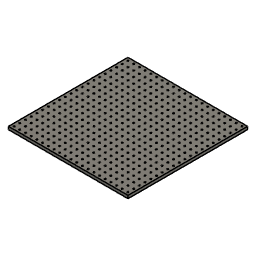
Robot base (Autodesk Fusion 360 design; units mm, degrees)
Autodesk Fusion 360 part; units mm, degrees
sketch "Sketch1" plane through (0, 0, 0) normal (0, 1, 0) x (1, 0, 0) in component "RobotPlatformBase"
  line L0 (-105, 105) -> (105, 105)
  line L1 (105, 105) -> (105, -105)
  line L2 (105, -105) -> (-105, -105)
  line L3 (-105, -105) -> (-105, 105)
  line L4 (-105, -105) -> (105, 105) construction
  dimension "d1" = 210
  constraint horizontal L0
  constraint vertical L1
  constraint horizontal L2
  constraint vertical L3
  constraint midpoint origin L4
  constraint equal L0 L3
  measures "d1" distance of L0.start L0.end
extrude "Extrude1" add sketch "Sketch1" along normal blind 5 in component "RobotPlatformBase"
sketch "Sketch2" plane through (0, 5, 0) normal (0, 1, 0) x (-1, 0, 0) in component "RobotPlatformBase"
  line L0 (105, 105) -> (-105, 105)
  line L1 (-105, 105) -> (-105, -105)
  line L2 (-105, -105) -> (105, -105)
  line L3 (105, -105) -> (105, 105)
  circle A0 centre (100, -100) radius 1.35
  circle A1 centre (90, -100) radius 1.35
  circle A2 centre (80, -100) radius 1.35
  circle A3 centre (70, -100) radius 1.35
  circle A4 centre (60, -100) radius 1.35
  circle A5 centre (50, -100) radius 1.35
  circle A6 centre (40, -100) radius 1.35
  circle A7 centre (30, -100) radius 1.35
  circle A8 centre (20, -100) radius 1.35
  circle A9 centre (10, -100) radius 1.35
  circle A10 centre (0, -100) radius 1.35
  circle A11 centre (-10, -100) radius 1.35
  circle A12 centre (-20, -100) radius 1.35
  circle A13 centre (-30, -100) radius 1.35
  circle A14 centre (-40, -100) radius 1.35
  circle A15 centre (-50, -100) radius 1.35
  circle A16 centre (-60, -100) radius 1.35
  circle A17 centre (-70, -100) radius 1.35
  circle A18 centre (-80, -100) radius 1.35
  circle A19 centre (-90, -100) radius 1.35
  circle A20 centre (100, -90) radius 1.35
  circle A21 centre (90, -90) radius 1.35
  circle A22 centre (80, -90) radius 1.35
  circle A23 centre (70, -90) radius 1.35
  circle A24 centre (60, -90) radius 1.35
  circle A25 centre (50, -90) radius 1.35
  circle A26 centre (40, -90) radius 1.35
  circle A27 centre (30, -90) radius 1.35
  circle A28 centre (20, -90) radius 1.35
  circle A29 centre (10, -90) radius 1.35
  circle A30 centre (0, -90) radius 1.35
  circle A31 centre (-10, -90) radius 1.35
  circle A32 centre (-20, -90) radius 1.35
  circle A33 centre (-30, -90) radius 1.35
  circle A34 centre (-40, -90) radius 1.35
  circle A35 centre (-50, -90) radius 1.35
  circle A36 centre (-60, -90) radius 1.35
  circle A37 centre (-70, -90) radius 1.35
  circle A38 centre (-80, -90) radius 1.35
  circle A39 centre (-90, -90) radius 1.35
  circle A40 centre (100, -80) radius 1.35
  circle A41 centre (90, -80) radius 1.35
  circle A42 centre (80, -80) radius 1.35
  circle A43 centre (70, -80) radius 1.35
  circle A44 centre (60, -80) radius 1.35
  circle A45 centre (50, -80) radius 1.35
  circle A46 centre (40, -80) radius 1.35
  circle A47 centre (30, -80) radius 1.35
  circle A48 centre (20, -80) radius 1.35
  circle A49 centre (10, -80) radius 1.35
  circle A50 centre (0, -80) radius 1.35
  circle A51 centre (-10, -80) radius 1.35
  circle A52 centre (-20, -80) radius 1.35
  circle A53 centre (-30, -80) radius 1.35
  circle A54 centre (-40, -80) radius 1.35
  circle A55 centre (-50, -80) radius 1.35
  circle A56 centre (-60, -80) radius 1.35
  circle A57 centre (-70, -80) radius 1.35
  circle A58 centre (-80, -80) radius 1.35
  circle A59 centre (-90, -80) radius 1.35
  circle A60 centre (100, -70) radius 1.35
  circle A61 centre (90, -70) radius 1.35
  circle A62 centre (80, -70) radius 1.35
  circle A63 centre (70, -70) radius 1.35
  circle A64 centre (60, -70) radius 1.35
  circle A65 centre (50, -70) radius 1.35
  circle A66 centre (40, -70) radius 1.35
  circle A67 centre (30, -70) radius 1.35
  circle A68 centre (20, -70) radius 1.35
  circle A69 centre (10, -70) radius 1.35
  circle A70 centre (0, -70) radius 1.35
  circle A71 centre (-10, -70) radius 1.35
  circle A72 centre (-20, -70) radius 1.35
  circle A73 centre (-30, -70) radius 1.35
  circle A74 centre (-40, -70) radius 1.35
  circle A75 centre (-50, -70) radius 1.35
  circle A76 centre (-60, -70) radius 1.35
  circle A77 centre (-70, -70) radius 1.35
  circle A78 centre (-80, -70) radius 1.35
  circle A79 centre (-90, -70) radius 1.35
  circle A80 centre (100, -60) radius 1.35
  circle A81 centre (90, -60) radius 1.35
  circle A82 centre (80, -60) radius 1.35
  circle A83 centre (70, -60) radius 1.35
  circle A84 centre (60, -60) radius 1.35
  circle A85 centre (50, -60) radius 1.35
  circle A86 centre (40, -60) radius 1.35
  circle A87 centre (30, -60) radius 1.35
  circle A88 centre (20, -60) radius 1.35
  circle A89 centre (10, -60) radius 1.35
  circle A90 centre (0, -60) radius 1.35
  circle A91 centre (-10, -60) radius 1.35
  circle A92 centre (-20, -60) radius 1.35
  circle A93 centre (-30, -60) radius 1.35
  circle A94 centre (-40, -60) radius 1.35
  circle A95 centre (-50, -60) radius 1.35
  circle A96 centre (-60, -60) radius 1.35
  circle A97 centre (-70, -60) radius 1.35
  circle A98 centre (-80, -60) radius 1.35
  circle A99 centre (-90, -60) radius 1.35
  circle A100 centre (100, -50) radius 1.35
  circle A101 centre (90, -50) radius 1.35
  circle A102 centre (80, -50) radius 1.35
  circle A103 centre (70, -50) radius 1.35
  circle A104 centre (60, -50) radius 1.35
  circle A105 centre (50, -50) radius 1.35
  circle A106 centre (40, -50) radius 1.35
  circle A107 centre (30, -50) radius 1.35
  circle A108 centre (20, -50) radius 1.35
  circle A109 centre (10, -50) radius 1.35
  circle A110 centre (0, -50) radius 1.35
  circle A111 centre (-10, -50) radius 1.35
  circle A112 centre (-20, -50) radius 1.35
  circle A113 centre (-30, -50) radius 1.35
  circle A114 centre (-40, -50) radius 1.35
  circle A115 centre (-50, -50) radius 1.35
  circle A116 centre (-60, -50) radius 1.35
  circle A117 centre (-70, -50) radius 1.35
  circle A118 centre (-80, -50) radius 1.35
  circle A119 centre (-90, -50) radius 1.35
  circle A120 centre (100, -40) radius 1.35
  circle A121 centre (90, -40) radius 1.35
  circle A122 centre (80, -40) radius 1.35
  circle A123 centre (70, -40) radius 1.35
  circle A124 centre (60, -40) radius 1.35
  circle A125 centre (50, -40) radius 1.35
  circle A126 centre (40, -40) radius 1.35
  circle A127 centre (30, -40) radius 1.35
  circle A128 centre (20, -40) radius 1.35
  circle A129 centre (10, -40) radius 1.35
  circle A130 centre (0, -40) radius 1.35
  circle A131 centre (-10, -40) radius 1.35
  circle A132 centre (-20, -40) radius 1.35
  circle A133 centre (-30, -40) radius 1.35
  circle A134 centre (-40, -40) radius 1.35
  circle A135 centre (-50, -40) radius 1.35
  circle A136 centre (-60, -40) radius 1.35
  circle A137 centre (-70, -40) radius 1.35
  circle A138 centre (-80, -40) radius 1.35
  circle A139 centre (-90, -40) radius 1.35
  circle A140 centre (100, -30) radius 1.35
  circle A141 centre (90, -30) radius 1.35
  circle A142 centre (80, -30) radius 1.35
  circle A143 centre (70, -30) radius 1.35
  circle A144 centre (60, -30) radius 1.35
  circle A145 centre (50, -30) radius 1.35
  circle A146 centre (40, -30) radius 1.35
  circle A147 centre (30, -30) radius 1.35
  circle A148 centre (20, -30) radius 1.35
  circle A149 centre (10, -30) radius 1.35
  circle A150 centre (0, -30) radius 1.35
  circle A151 centre (-10, -30) radius 1.35
  circle A152 centre (-20, -30) radius 1.35
  circle A153 centre (-30, -30) radius 1.35
  circle A154 centre (-40, -30) radius 1.35
  circle A155 centre (-50, -30) radius 1.35
  circle A156 centre (-60, -30) radius 1.35
  circle A157 centre (-70, -30) radius 1.35
  circle A158 centre (-80, -30) radius 1.35
  circle A159 centre (-90, -30) radius 1.35
  circle A160 centre (100, -20) radius 1.35
  circle A161 centre (90, -20) radius 1.35
  circle A162 centre (80, -20) radius 1.35
  circle A163 centre (70, -20) radius 1.35
  circle A164 centre (60, -20) radius 1.35
  circle A165 centre (50, -20) radius 1.35
  circle A166 centre (40, -20) radius 1.35
  circle A167 centre (30, -20) radius 1.35
  circle A168 centre (20, -20) radius 1.35
  circle A169 centre (10, -20) radius 1.35
  circle A170 centre (0, -20) radius 1.35
  circle A171 centre (-10, -20) radius 1.35
  circle A172 centre (-20, -20) radius 1.35
  circle A173 centre (-30, -20) radius 1.35
  circle A174 centre (-40, -20) radius 1.35
  circle A175 centre (-50, -20) radius 1.35
  circle A176 centre (-60, -20) radius 1.35
  circle A177 centre (-70, -20) radius 1.35
  circle A178 centre (-80, -20) radius 1.35
  circle A179 centre (-90, -20) radius 1.35
  circle A180 centre (100, -10) radius 1.35
  circle A181 centre (90, -10) radius 1.35
  circle A182 centre (80, -10) radius 1.35
  circle A183 centre (70, -10) radius 1.35
  circle A184 centre (60, -10) radius 1.35
  circle A185 centre (50, -10) radius 1.35
  circle A186 centre (40, -10) radius 1.35
  circle A187 centre (30, -10) radius 1.35
  circle A188 centre (20, -10) radius 1.35
  circle A189 centre (10, -10) radius 1.35
  circle A190 centre (0, -10) radius 1.35
  circle A191 centre (-10, -10) radius 1.35
  circle A192 centre (-20, -10) radius 1.35
  circle A193 centre (-30, -10) radius 1.35
  circle A194 centre (-40, -10) radius 1.35
  circle A195 centre (-50, -10) radius 1.35
  circle A196 centre (-60, -10) radius 1.35
  circle A197 centre (-70, -10) radius 1.35
  circle A198 centre (-80, -10) radius 1.35
  circle A199 centre (-90, -10) radius 1.35
  circle A200 centre (100, 0) radius 1.35
  circle A201 centre (90, 0) radius 1.35
  circle A202 centre (80, 0) radius 1.35
  circle A203 centre (70, 0) radius 1.35
  circle A204 centre (60, 0) radius 1.35
  circle A205 centre (50, 0) radius 1.35
  circle A206 centre (40, 0) radius 1.35
  circle A207 centre (30, 0) radius 1.35
  circle A208 centre (20, 0) radius 1.35
  circle A209 centre (10, 0) radius 1.35
  circle A210 centre (0, 0) radius 1.35
  circle A211 centre (-10, 0) radius 1.35
  circle A212 centre (-20, 0) radius 1.35
  circle A213 centre (-30, 0) radius 1.35
  circle A214 centre (-40, 0) radius 1.35
  circle A215 centre (-50, 0) radius 1.35
  circle A216 centre (-60, 0) radius 1.35
  circle A217 centre (-70, 0) radius 1.35
  circle A218 centre (-80, 0) radius 1.35
  circle A219 centre (-90, 0) radius 1.35
  circle A220 centre (100, 10) radius 1.35
  circle A221 centre (90, 10) radius 1.35
  circle A222 centre (80, 10) radius 1.35
  circle A223 centre (70, 10) radius 1.35
  circle A224 centre (60, 10) radius 1.35
  circle A225 centre (50, 10) radius 1.35
  circle A226 centre (40, 10) radius 1.35
  circle A227 centre (30, 10) radius 1.35
  circle A228 centre (20, 10) radius 1.35
  circle A229 centre (10, 10) radius 1.35
  circle A230 centre (0, 10) radius 1.35
  circle A231 centre (-10, 10) radius 1.35
  circle A232 centre (-20, 10) radius 1.35
  circle A233 centre (-30, 10) radius 1.35
  circle A234 centre (-40, 10) radius 1.35
  circle A235 centre (-50, 10) radius 1.35
  circle A236 centre (-60, 10) radius 1.35
  circle A237 centre (-70, 10) radius 1.35
  circle A238 centre (-80, 10) radius 1.35
  circle A239 centre (-90, 10) radius 1.35
  circle A240 centre (100, 20) radius 1.35
  circle A241 centre (90, 20) radius 1.35
  circle A242 centre (80, 20) radius 1.35
  circle A243 centre (70, 20) radius 1.35
  circle A244 centre (60, 20) radius 1.35
  circle A245 centre (50, 20) radius 1.35
  circle A246 centre (40, 20) radius 1.35
  circle A247 centre (30, 20) radius 1.35
  circle A248 centre (20, 20) radius 1.35
  circle A249 centre (10, 20) radius 1.35
  circle A250 centre (0, 20) radius 1.35
  circle A251 centre (-10, 20) radius 1.35
  circle A252 centre (-20, 20) radius 1.35
  circle A253 centre (-30, 20) radius 1.35
  circle A254 centre (-40, 20) radius 1.35
  circle A255 centre (-50, 20) radius 1.35
  circle A256 centre (-60, 20) radius 1.35
  circle A257 centre (-70, 20) radius 1.35
  circle A258 centre (-80, 20) radius 1.35
  circle A259 centre (-90, 20) radius 1.35
  circle A260 centre (100, 30) radius 1.35
  circle A261 centre (90, 30) radius 1.35
  circle A262 centre (80, 30) radius 1.35
  circle A263 centre (70, 30) radius 1.35
  circle A264 centre (60, 30) radius 1.35
  circle A265 centre (50, 30) radius 1.35
  circle A266 centre (40, 30) radius 1.35
  circle A267 centre (30, 30) radius 1.35
  circle A268 centre (20, 30) radius 1.35
  circle A269 centre (10, 30) radius 1.35
  circle A270 centre (0, 30) radius 1.35
  circle A271 centre (-10, 30) radius 1.35
  circle A272 centre (-20, 30) radius 1.35
  circle A273 centre (-30, 30) radius 1.35
  circle A274 centre (-40, 30) radius 1.35
  circle A275 centre (-50, 30) radius 1.35
  circle A276 centre (-60, 30) radius 1.35
  circle A277 centre (-70, 30) radius 1.35
  circle A278 centre (-80, 30) radius 1.35
  circle A279 centre (-90, 30) radius 1.35
  circle A280 centre (100, 40) radius 1.35
  circle A281 centre (90, 40) radius 1.35
  circle A282 centre (80, 40) radius 1.35
  circle A283 centre (70, 40) radius 1.35
  circle A284 centre (60, 40) radius 1.35
  circle A285 centre (50, 40) radius 1.35
  circle A286 centre (40, 40) radius 1.35
  circle A287 centre (30, 40) radius 1.35
  circle A288 centre (20, 40) radius 1.35
  circle A289 centre (10, 40) radius 1.35
  circle A290 centre (0, 40) radius 1.35
  circle A291 centre (-10, 40) radius 1.35
  circle A292 centre (-20, 40) radius 1.35
  circle A293 centre (-30, 40) radius 1.35
  circle A294 centre (-40, 40) radius 1.35
  circle A295 centre (-50, 40) radius 1.35
  circle A296 centre (-60, 40) radius 1.35
  circle A297 centre (-70, 40) radius 1.35
  circle A298 centre (-80, 40) radius 1.35
  circle A299 centre (-90, 40) radius 1.35
  circle A300 centre (100, 50) radius 1.35
  circle A301 centre (90, 50) radius 1.35
  circle A302 centre (80, 50) radius 1.35
  circle A303 centre (70, 50) radius 1.35
  circle A304 centre (60, 50) radius 1.35
  circle A305 centre (50, 50) radius 1.35
  circle A306 centre (40, 50) radius 1.35
  circle A307 centre (30, 50) radius 1.35
  circle A308 centre (20, 50) radius 1.35
  circle A309 centre (10, 50) radius 1.35
  circle A310 centre (0, 50) radius 1.35
  circle A311 centre (-10, 50) radius 1.35
  circle A312 centre (-20, 50) radius 1.35
  circle A313 centre (-30, 50) radius 1.35
  circle A314 centre (-40, 50) radius 1.35
  circle A315 centre (-50, 50) radius 1.35
  circle A316 centre (-60, 50) radius 1.35
  circle A317 centre (-70, 50) radius 1.35
  circle A318 centre (-80, 50) radius 1.35
  circle A319 centre (-90, 50) radius 1.35
  circle A320 centre (100, 60) radius 1.35
  circle A321 centre (90, 60) radius 1.35
  circle A322 centre (80, 60) radius 1.35
  circle A323 centre (70, 60) radius 1.35
  circle A324 centre (60, 60) radius 1.35
  circle A325 centre (50, 60) radius 1.35
  circle A326 centre (40, 60) radius 1.35
  circle A327 centre (30, 60) radius 1.35
  circle A328 centre (20, 60) radius 1.35
  circle A329 centre (10, 60) radius 1.35
  circle A330 centre (0, 60) radius 1.35
  circle A331 centre (-10, 60) radius 1.35
  circle A332 centre (-20, 60) radius 1.35
  circle A333 centre (-30, 60) radius 1.35
  circle A334 centre (-40, 60) radius 1.35
  circle A335 centre (-50, 60) radius 1.35
  circle A336 centre (-60, 60) radius 1.35
  circle A337 centre (-70, 60) radius 1.35
  circle A338 centre (-80, 60) radius 1.35
  circle A339 centre (-90, 60) radius 1.35
  circle A340 centre (100, 70) radius 1.35
  circle A341 centre (90, 70) radius 1.35
  circle A342 centre (80, 70) radius 1.35
  circle A343 centre (70, 70) radius 1.35
  circle A344 centre (60, 70) radius 1.35
  circle A345 centre (50, 70) radius 1.35
  circle A346 centre (40, 70) radius 1.35
  circle A347 centre (30, 70) radius 1.35
  circle A348 centre (20, 70) radius 1.35
  circle A349 centre (10, 70) radius 1.35
  circle A350 centre (0, 70) radius 1.35
  circle A351 centre (-10, 70) radius 1.35
  circle A352 centre (-20, 70) radius 1.35
  circle A353 centre (-30, 70) radius 1.35
  circle A354 centre (-40, 70) radius 1.35
  circle A355 centre (-50, 70) radius 1.35
  circle A356 centre (-60, 70) radius 1.35
  circle A357 centre (-70, 70) radius 1.35
  circle A358 centre (-80, 70) radius 1.35
  circle A359 centre (-90, 70) radius 1.35
  circle A360 centre (100, 80) radius 1.35
  circle A361 centre (90, 80) radius 1.35
  circle A362 centre (80, 80) radius 1.35
  circle A363 centre (70, 80) radius 1.35
  circle A364 centre (60, 80) radius 1.35
  circle A365 centre (50, 80) radius 1.35
  circle A366 centre (40, 80) radius 1.35
  circle A367 centre (30, 80) radius 1.35
  circle A368 centre (20, 80) radius 1.35
  circle A369 centre (10, 80) radius 1.35
  circle A370 centre (0, 80) radius 1.35
  circle A371 centre (-10, 80) radius 1.35
  circle A372 centre (-20, 80) radius 1.35
  circle A373 centre (-30, 80) radius 1.35
  circle A374 centre (-40, 80) radius 1.35
  circle A375 centre (-50, 80) radius 1.35
  circle A376 centre (-60, 80) radius 1.35
  circle A377 centre (-70, 80) radius 1.35
  circle A378 centre (-80, 80) radius 1.35
  circle A379 centre (-90, 80) radius 1.35
  circle A380 centre (100, 90) radius 1.35
  circle A381 centre (90, 90) radius 1.35
  circle A382 centre (80, 90) radius 1.35
  circle A383 centre (70, 90) radius 1.35
  circle A384 centre (60, 90) radius 1.35
  circle A385 centre (50, 90) radius 1.35
  circle A386 centre (40, 90) radius 1.35
  circle A387 centre (30, 90) radius 1.35
  circle A388 centre (20, 90) radius 1.35
  circle A389 centre (10, 90) radius 1.35
  circle A390 centre (0, 90) radius 1.35
  circle A391 centre (-10, 90) radius 1.35
  circle A392 centre (-20, 90) radius 1.35
  circle A393 centre (-30, 90) radius 1.35
  circle A394 centre (-40, 90) radius 1.35
  circle A395 centre (-50, 90) radius 1.35
  circle A396 centre (-60, 90) radius 1.35
  circle A397 centre (-70, 90) radius 1.35
  circle A398 centre (-80, 90) radius 1.35
  circle A399 centre (-90, 90) radius 1.35
  circle A400 centre (-100, -100) radius 1.35
  circle A401 centre (-100, -90) radius 1.35
  circle A402 centre (-100, -80) radius 1.35
  circle A403 centre (-100, -70) radius 1.35
  circle A404 centre (-100, -60) radius 1.35
  circle A405 centre (-100, -50) radius 1.35
  circle A406 centre (-100, -40) radius 1.35
  circle A407 centre (-100, -30) radius 1.35
  circle A408 centre (-100, -20) radius 1.35
  circle A409 centre (-100, -10) radius 1.35
  circle A410 centre (-100, 0) radius 1.35
  circle A411 centre (-100, 10) radius 1.35
  circle A412 centre (-100, 20) radius 1.35
  circle A413 centre (-100, 30) radius 1.35
  circle A414 centre (-100, 40) radius 1.35
  circle A415 centre (-100, 50) radius 1.35
  circle A416 centre (-100, 60) radius 1.35
  circle A417 centre (-100, 70) radius 1.35
  circle A418 centre (-100, 80) radius 1.35
  circle A419 centre (-100, 90) radius 1.35
  circle A420 centre (100, 100) radius 1.35
  circle A421 centre (90, 100) radius 1.35
  circle A422 centre (80, 100) radius 1.35
  circle A423 centre (70, 100) radius 1.35
  circle A424 centre (60, 100) radius 1.35
  circle A425 centre (50, 100) radius 1.35
  circle A426 centre (40, 100) radius 1.35
  circle A427 centre (30, 100) radius 1.35
  circle A428 centre (20, 100) radius 1.35
  circle A429 centre (10, 100) radius 1.35
  circle A430 centre (0, 100) radius 1.35
  circle A431 centre (-10, 100) radius 1.35
  circle A432 centre (-20, 100) radius 1.35
  circle A433 centre (-30, 100) radius 1.35
  circle A434 centre (-40, 100) radius 1.35
  circle A435 centre (-50, 100) radius 1.35
  circle A436 centre (-60, 100) radius 1.35
  circle A437 centre (-70, 100) radius 1.35
  circle A438 centre (-80, 100) radius 1.35
  circle A439 centre (-90, 100) radius 1.35
  circle A440 centre (-100, 100) radius 1.35
  dimension "d4" = 2.7
  dimension "d7" = -10
  dimension "d8" = 10
  constraint coincident A210.centre origin
  measures "d4" diameter of A0
extrude "Extrude2" cut sketch "Sketch2" against normal up to surface (5 mm away) contours A0 | A1 | A2 | A3 | A4 | A5 | A6 | A7 | A8 | A9 | A10 | A11 | A12 | A13 | A14 | A15 | A16 | A17 | A18 | A19 | A20 | A21 | A22 | A23 | A24 | A25 | A26 | A27 | A28 | A29 | A30 | A31 | A32 | A33 | A34 | A35 | A36 | A37 | A38 | A39 | A40 | A41 | A42 | A43 | A44 | A45 | A46 | A47 | A48 | A49 | A50 | A51 | A52 | A53 | A54 | A55 | A56 | A57 | A58 | A59 | A60 | A61 | A62 | A63 | A64 | A65 | A66 | A67 | A68 | A69 | A70 | A71 | A72 | A73 | A74 | A75 | A76 | A77 | A78 | A79 | A80 | A81 | A82 | A83 | A84 | A85 | A86 | A87 | A88 | A89 | A90 | A91 | A92 | A93 | A94 | A95 | A96 | A97 | A98 | A99 | A100 | A101 | A102 | A103 | A104 | A105 | A106 | A107 | A108 | A109 | A110 | A111 | A112 | A113 | A114 | A115 | A116 | A117 | A118 | A119 | A120 | A121 | A122 | A123 | A124 | A125 | A126 | A127 | A128 | A129 | A130 | A131 | A132 | A133 | A134 | A135 | A136 | A137 | A138 | A139 | A140 | A141 | A142 | A143 | A144 | A145 | A146 | A147 | A148 | A149 | A150 | A151 | A152 | A153 | A154 | A155 | A156 | A157 | A158 | A159 | A160 | A161 | A162 | A163 | A164 | A165 | A166 | A167 | A168 | A169 | A170 | A171 | A172 | A173 | A174 | A175 | A176 | A177 | A178 | A179 | A180 | A181 | A182 | A183 | A184 | A185 | A186 | A187 | A188 | A189 | A190 | A191 | A192 | A193 | A194 | A195 | A196 | A197 | A198 | A199 | A200 | A201 | A202 | A203 | A204 | A205 | A206 | A207 | A208 | A209 | A210 | A211 | A212 | A213 | A214 | A215 | A216 | A217 | A218 | A219 | A220 | A221 | A222 | A223 | A224 | A225 | A226 | A227 | A228 | A229 | A230 | A231 | A232 | A233 | A234 | A235 | A236 | A237 | A238 | A239 | A240 | A241 | A242 | A243 | A244 | A245 | A246 | A247 | A248 | A249 | A250 | A251 | A252 | A253 | A254 | A255 | A256 | A257 | A258 | A259 | A260 | A261 | A262 | A263 | A264 | A265 | A266 | A267 | A268 | A269 | A270 | A271 | A272 | A273 | A274 | A275 | A276 | A277 | A278 | A279 | A280 | A281 | A282 | A283 | A284 | A285 | A286 | A287 | A288 | A289 | A290 | A291 | A292 | A293 | A294 | A295 | A296 | A297 | A298 | A299 | A300 | A301 | A302 | A303 | A304 | A305 | A306 | A307 | A308 | A309 | A310 | A311 | A312 | A313 | A314 | A315 | A316 | A317 | A318 | A319 | A320 | A321 | A322 | A323 | A324 | A325 | A326 | A327 | A328 | A329 | A330 | A331 | A332 | A333 | A334 | A335 | A336 | A337 | A338 | A339 | A340 | A341 | A342 | A343 | A344 | A345 | A346 | A347 | A348 | A349 | A350 | A351 | A352 | A353 | A354 | A355 | A356 | A357 | A358 | A359 | A360 | A361 | A362 | A363 | A364 | A365 | A366 | A367 | A368 | A369 | A370 | A371 | A372 | A373 | A374 | A375 | A376 | A377 | A378 | A379 | A380 | A381 | A382 | A383 | A384 | A385 | A386 | A387 | A388 | A389 | A390 | A391 | A392 | A393 | A394 | A395 | A396 | A397 | A398 | A399 | A400 | A401 | A402 | A403 | A404 | A405 | A406 | A407 | A408 | A409 | A410 | A411 | A412 | A413 | A414 | A415 | A416 | A417 | A418 | A419 | A420 | A421 | A422 | A423 | A424 | A425 | A426 | A427 | A428 | A429 | A430 | A431 | A432 | A433 | A434 | A435 | A436 | A437 | A438 | A439 | A440 in component "RobotPlatformBase"
component "RobotPlatformBase" placed x (1, 0, 0) y (0, 1, 0) z (0, 0, 1) at (0, 0, 0)
